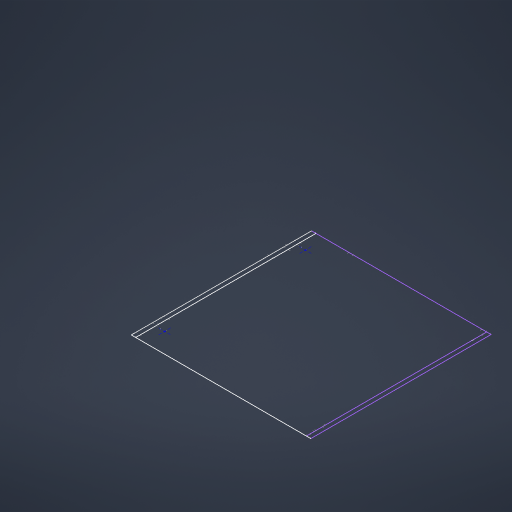
# Autodesk Inventor part: Деталь1
Saved by Autodesk Inventor 2023.4 (Build 274418000, 418)
## iProperties
Created: 2026-09-26
Part Number: Деталь1
Material: Типовые
Document SubType Name: Modeling
Designer: desig
Density: 1 g/cm^3
Appearance: По умолчанию
Author: desig
Autodesk Inventor part; units mm, degrees
ref_plane "YZ Plane" through (0, 0, 0) normal (1, 0, 0) x (0, 1, 0)
ref_plane "XZ Plane" through (0, 0, 0) normal (0, 1, 0) x (-1, 0, 0)
ref_plane "XY Plane" through (0, 0, 0) normal (0, 0, 1) x (1, 0, 0)
sketch "Эскиз1" plane through (0, 0, 0) normal (0, 1, 0) x (-1, 0, 0)
  line L0 (0, 0) -> (-16, 0)
  line L1 (-16, 0) -> (-16, -655.604)
  line L2 (-16, -655.604) -> (0, -655.604)
  line L3 (0, -655.604) -> (0, 0)
  line L4 (-636.8602, 0) -> (-652.8602, 0)
  line L5 (-652.8602, 0) -> (-652.8602, -655.604)
  line L6 (-652.8602, -655.604) -> (-636.8602, -655.604)
  line L7 (-636.8602, -655.604) -> (-636.8602, 0)
  line L8 (-16, -655.604) -> (-636.8602, -655.604)
  line L9 (-16, 0) -> (-636.8602, 0)
  dimension "d0" = 16
  dimension "d1" = 16
  dimension "d46" = 655.604
  dimension "d47" = 652.86
  constraints: 20 end point, 4 parallel, 3 horizontal, 3 perpendicular, 2 point on line
  measures "d0" distance of L1.end L2.end
  measures "d1" distance of L5.end L6.end
  measures "d46" distance of L2.end L0.start
  measures "d47" distance between parallel lines of L5 L3
extrude "Выдавливание1" add sketch "Эскиз1" along normal blind 500 contours L3 L2 L1 L0
extrude "Выдавливание2" add sketch "Эскиз1" against normal blind 16 from surface at 500 separate body contours L1 L8 L7 L9
extrude "Выдавливание3" add sketch "Эскиз1" along normal blind 16 separate body contours L1 L8 L7 L9
extrude "Выдавливание4" add sketch "Эскиз1" along normal up to surface (500 mm away) separate body contours L7 L6 L5 L4
sketch "DrillingSketch_1" plane through (636.8602, 484, 0) normal (1, 0, 0) x (0, 0, -1)
  line L0 (655.604, 0) -> (0, 0) projected
  line L1 (655.604, 0) -> (655.604, 16) projected
  line L2 (655.604, 16) -> (0, 16) projected
  line L3 (0, 0) -> (0, 16) projected
  line L4 (655.604, 8) -> (0, 8) construction
  line L5 (327.802, 8) -> (327.802, -12) construction
  point P0 (583.802, 8)
  point P1 (71.802, 8)
  point P2 (551.802, 8)
  point P3 (103.802, 8)
  dimension "d5" = 16
  dimension "Минимальный_отступ_присадки_от_кромки_Каркас" = 70
  dimension "Long_edge_1" = 655.604
  dimension "Расстояние_между_точками" = 512
  dimension "d733" = 32
  constraints: 5 point on line, 4 end point, 4 midpoint, 2 symmetric about line, 1 perpendicular
  measures "Long_edge_1" distance of L4.start L4.end
  measures "Расстояние_между_точками" distance of point (71.802, 8) point (583.802, 8)
  measures "d733" distance of point (583.802, 8) point (551.802, 8)
sketch "DrillingSketch_2" plane through (16, 0, -655.604) normal (-1, 0, 0) x (0, 0, 1)
  line L0 (0, 0) -> (655.604, 0) projected
  line L1 (655.604, 0) -> (655.604, 16) projected
  line L2 (0, 16) -> (655.604, 16) projected
  line L3 (0, 0) -> (0, 16) projected
  line L4 (655.604, 8) -> (0, 8) construction
  line L5 (327.802, 8) -> (327.802, -12) construction
  point P0 (583.802, 8)
  point P1 (71.802, 8)
  point P2 (551.802, 8)
  point P3 (103.802, 8)
  dimension "Минимальный_отступ_присадки_от_кромки_Каркас" = 70
  dimension "Long_edge_2" = 655.604
  dimension "Расстояние_между_точками_2" = 512
  dimension "d736" = 32
  constraints: 5 point on line, 4 end point, 4 midpoint, 2 symmetric about line, 1 perpendicular
  measures "Long_edge_2" distance of L4.start L4.end
  measures "Расстояние_между_точками_2" distance of point (71.802, 8) point (583.802, 8)
  measures "d736" distance of point (583.802, 8) point (551.802, 8)
sketch "DrawerSketch_1" plane through (16, 484, -655.604) normal (-1, 0, 0) x (0, 0, 1)
  line L0 (655.604, 0) -> (0, 0) projected
  line L1 (655.604, 16) -> (655.604, 0) projected
  line L2 (655.604, 16) -> (0, 16) projected
  line L3 (0, 0) -> (0, 16) projected
  line L4 (655.604, 8) -> (0, 8) construction
  line L5 (327.802, 8) -> (327.802, -12) construction
  point P0 (631.802, 8)
  point P1 (23.802, 8)
  point P2 (599.802, 8)
  point P3 (55.802, 8)
  dimension "d46" = 655.604
  dimension "d47" = 652.86
  dimension "Минимальный_отступ_присадки_от_кромки_Ящик" = 20
  dimension "Long_edge_1_2" = 655.604
  dimension "Расстояние_между_точками_3" = 608
  dimension "d739" = 32
  constraints: 5 point on line, 4 end point, 4 midpoint, 2 symmetric about line, 1 perpendicular
  measures "Long_edge_1_2" distance of L4.start L4.end
  measures "Расстояние_между_точками_3" distance of point (23.802, 8) point (631.802, 8)
  measures "d739" distance of point (631.802, 8) point (599.802, 8)
sketch "DrawerSketch_2" plane through (636.8602, 0, 0) normal (1, 0, 0) x (0, 0, -1)
  line L0 (0, 0) -> (655.604, 0) projected
  line L1 (655.604, 0) -> (655.604, 16) projected
  line L2 (0, 16) -> (655.604, 16) projected
  line L3 (0, 0) -> (0, 16) projected
  line L4 (655.604, 8) -> (0, 8) construction
  line L5 (327.802, 8) -> (327.802, -12) construction
  point P0 (631.802, 8)
  point P1 (23.802, 8)
  point P2 (599.802, 8)
  point P3 (55.802, 8)
  dimension "d46" = 655.604
  dimension "d47" = 652.86
  dimension "Минимальный_отступ_присадки_от_кромки_Ящик" = 20
  dimension "Long_edge_2_2" = 655.604
  dimension "Расстояние_между_точками_4" = 608
  dimension "d742" = 32
  constraints: 5 point on line, 4 end point, 4 midpoint, 2 symmetric about line, 1 perpendicular
  measures "Long_edge_2_2" distance of L4.start L4.end
  measures "Расстояние_между_точками_4" distance of point (23.802, 8) point (631.802, 8)
  measures "d742" distance of point (631.802, 8) point (599.802, 8)
hole "Stiajka outer 8x34" at (16, 492, -23.802) at (16, 492, -631.802) direction (1, 0, 0) diameter 8 depth 34 bodies 1 2 3 4
hole "Stiajka outer 5x13" at (16, 492, -23.802) at (16, 492, -631.802) direction (-1, 0, 0) diameter 5 depth 13 bodies 1 2 3 4
hole "Stiajka inner 8x10" at (16, 492, -55.802) at (16, 492, -599.802) direction (-1, 0, 0) diameter 8 depth 10 bodies 1 2 3 4
hole "Stiajka inner 8x20" at (16, 492, -55.802) at (16, 492, -599.802) direction (1, 0, 0) diameter 8 depth 20 bodies 1 2 3 4
sketch "StiajkaSideSketch" plane through (16, 484, 0) normal (0, -1, 0) x (1, 0, 0)
  line L0 (0, -27.802) -> (0, -19.802) projected
  line L1 (34, -19.802) -> (34, -27.802) projected
  line L2 (0, -635.802) -> (0, -627.802) projected
  line L3 (34, -627.802) -> (34, -635.802) projected
  point P0 (34, -23.802)
  point P1 (34, -631.802)
  dimension "d46" = 655.604
  dimension "d47" = 652.86
  constraints: 2 midpoint
hole "Stiajka cup" at (50, 484, -23.802) at (50, 484, -631.802) direction (0, 1, 0) diameter 15 depth 12.5 bodies 1 2 3 4
hole "Stiajka outer 8x34 2" at (636.8602, 8, -631.802) at (636.8602, 8, -23.802) direction (-1, 0, 0) diameter 8 depth 34 bodies 1 2 3 4
hole "Stiajka outer 5x13 2" at (636.8602, 8, -631.802) at (636.8602, 8, -23.802) direction (1, 0, 0) diameter 5 depth 13 bodies 1 2 3 4
hole "Stiajka inner 8x10 2" at (636.8602, 8, -599.802) at (636.8602, 8, -55.802) direction (1, 0, 0) diameter 8 depth 10 bodies 1 2 3 4
hole "Stiajka inner 8x20 2" at (636.8602, 8, -599.802) at (636.8602, 8, -55.802) direction (-1, 0, 0) diameter 8 depth 20 bodies 1 2 3 4
sketch "StiajkaSideSketch_2" plane through (0, 0, 0) normal (0, -1, 0) x (1, 0, 0)
  line L0 (636.8602, -627.802) -> (636.8602, -635.802) projected
  line L1 (602.8602, -635.802) -> (602.8602, -627.802) projected
  line L2 (636.8602, -19.802) -> (636.8602, -27.802) projected
  line L3 (602.8602, -27.802) -> (602.8602, -19.802) projected
  point P0 (602.8602, -631.802)
  point P1 (602.8602, -23.802)
  dimension "d46" = 655.604
  dimension "d47" = 652.86
  constraints: 2 midpoint
hole "Stiajka cup 2" at (602.8602, 0, -631.802) at (602.8602, 0, -23.802) direction (0, 1, 0) diameter 15 depth 12.5 bodies 1 2 3 4
hole "Confirmat 5mm inward" at (636.8602, 492, -583.802) at (636.8602, 492, -327.802) at (636.8602, 492, -71.802) direction (1, 0, 0) diameter 5 depth 20 bodies 1 2 3 4
hole "Confirmat 3mm outward" at (636.8602, 492, -583.802) at (636.8602, 492, -327.802) at (636.8602, 492, -71.802) direction (-1, 0, 0) diameter 3 depth 50 bodies 1 2 3 4
hole "Stiajka outer 8x34 3" at (16, 8, -71.802) at (16, 8, -583.802) direction (1, 0, 0) diameter 8 depth 34 bodies 1 2 3 4
hole "Stiajka outer 5x13 3" at (16, 8, -71.802) at (16, 8, -583.802) direction (-1, 0, 0) diameter 5 depth 13 bodies 1 2 3 4
hole "Stiajka inner 8x10 3" at (16, 8, -103.802) at (16, 8, -551.802) direction (-1, 0, 0) diameter 8 depth 10 bodies 1 2 3 4
hole "Stiajka inner 8x20 3" at (16, 8, -103.802) at (16, 8, -551.802) direction (1, 0, 0) diameter 8 depth 20 bodies 1 2 3 4
sketch "StiajkaSideSketch_3" plane through (0, 0, 0) normal (0, -1, 0) x (1, 0, 0)
  line L0 (16, -75.802) -> (16, -67.802) projected
  line L1 (50, -67.802) -> (50, -75.802) projected
  line L2 (16, -587.802) -> (16, -579.802) projected
  line L3 (50, -579.802) -> (50, -587.802) projected
  point P0 (50, -71.802)
  point P1 (50, -583.802)
  dimension "d46" = 655.604
  dimension "d47" = 652.86
  constraints: 2 midpoint
hole "Stiajka cup 3" [suppressed]
sketch "Эскиз56" plane through (0, 16, 0) normal (0, 1, 0) x (1, 0, 0)
  point P0 (0, 0)
  point P1 (50, 67.802)
  point P2 (50, 579.802)
  dimension "d46" = 655.604
  dimension "d47" = 652.86
hole "Отверстие102" at (50, 16, -579.802) at (50, 16, -67.802) direction (0, -1, 0) diameter 15 depth 13 bodies 3
equation "\"d0\" = Толщина_каркаса"
equation "\"d1\" = Толщина_каркаса"
equation "\"d5\" = Толщина_каркаса"
equation "\"d7\" = Толщина_каркаса"
equation "\"Минимальный_отступ_присадки_от_кромки_Каркас\" = 70"
equation "\"Минимальный_отступ_присадки_от_кромки_Ящик\" = 20"
equation "\"d771\" = Стяжка_D"
equation "\"d776\" = Стяжка_h"
equation "\"d806\" = Стяжка_D"
equation "\"d811\" = Стяжка_h"
equation "\"d855\" = Стяжка_D"
equation "\"d860\" = Стяжка_h"
equation "\"d862\" = Стяжка_D"
equation "\"Толщина_каркаса\" = 16"
equation "\"Стяжка_D\" = 15"
equation "\"Стяжка_h\" = 12.5"
equation "\"Стяжка_D_резьбыШтока\" = 5"
equation "\"Стяжка_D_телаШтока\" = 8"
equation "\"Стяжка_резьбыШтока_Петля_h\" = 12.5"
equation "\"Стяжка_отступ\" = 34"
equation "\"Конфирмат_D_вПласть\" = 8"
equation "\"Конфирмат_D_вТорец\" = 5"
equation "\"Толщина_каркаса_ящика\" = 16"
equation "\"Шкант_D\" = 8"
equation "\"Полкодержатель_D\" = 5"
equation "\"Полкодержатель_смещение_от_низа_полки\" = 5"
equation "\"Петля_D_присадки\" = 35"
equation "\"M_Конфирмат_глубина_резьбы\" = 35"
equation "\"M_Конфирмат_D_вПласть\" = 5"
equation "\"M_Конфирмат_D_вТорец\" = 3"
equation "\"Толщина_задн_ст_Володя\" = 3"
equation "\"Толщина_дна_ящика_Володя\" = 6"
equation "\"Минимальное_расстояния_от_заднСт_ящика_до_заднСт\" = 25"
equation "\"Западание_кромки_полки_за_каркас\" = 5"
